Autodesk Fusion 360 part; units mm, degrees
(part 4 of 5)
  spline S202 degree 5 poles (32.0875, 34.5814) (32.0719, 34.5758) (32.0408, 34.5645) (31.9942, 34.5475) (31.9321, 34.5247) (31.8546, 34.496) (31.7774, 34.4669) (31.7004, 34.4376) (31.6235, 34.408) (31.5469, 34.3781) (31.4704, 34.348) (31.3942, 34.3176) (31.3181, 34.2869) (31.2423, 34.2559) (31.1666, 34.2246) (31.0912, 34.1931) (31.016, 34.1613) (30.941, 34.1291) (30.8662, 34.0967) (30.7916, 34.0641) (30.7172, 34.0311) (30.6563, 34.0037) (30.6103, 33.9829) (30.5792, 33.9687) (30.5628, 33.9613) (30.5612, 33.9605) knots -1 -1 -1 -1 -1 -1 -0.985714 -0.971429 -0.957143 -0.942857 -0.928571 -0.914286 -0.9 -0.885714 -0.871429 -0.857143 -0.842857 -0.828571 -0.814286 -0.8 -0.785714 -0.771429 -0.757143 -0.742857 -0.728571 -0.714286 -0.712736 -0.712736 -0.712736 -0.712736 -0.712736 -0.712736
  spline S203 degree 5 poles (-44.686, 9.5112) (-44.6878, 9.5109) (-44.7054, 9.5073) (-44.7389, 9.5005) (-44.7884, 9.4903) (-44.8537, 9.4766) (-44.9333, 9.4596) (-45.0128, 9.4422) (-45.0924, 9.4244) (-45.1719, 9.4063) (-45.2515, 9.3878) (-45.3311, 9.369) (-45.4106, 9.3498) (-45.4902, 9.3303) (-45.5698, 9.3105) (-45.6494, 9.2903) (-45.7289, 9.2697) (-45.8085, 9.2488) (-45.8881, 9.2276) (-45.9676, 9.206) (-46.0472, 9.1841) (-46.1267, 9.1619) (-46.1903, 9.1438) (-46.2381, 9.1301) (-46.2699, 9.121) (-46.2858, 9.1163) knots 0.712736 0.712736 0.712736 0.712736 0.712736 0.712736 0.714286 0.728571 0.742857 0.757143 0.771429 0.785714 0.8 0.814286 0.828571 0.842857 0.857143 0.871429 0.885714 0.9 0.914286 0.928571 0.942857 0.957143 0.971429 0.985714 1 1 1 1 1 1
  spline S204 degree 5 poles (-29.8528, -36.5279) (-29.8376, -36.5213) (-29.8073, -36.5081) (-29.7618, -36.4883) (-29.7012, -36.4616) (-29.6258, -36.4281) (-29.5505, -36.3942) (-29.4755, -36.3601) (-29.4006, -36.3258) (-29.326, -36.2911) (-29.2516, -36.2563) (-29.1774, -36.2211) (-29.1034, -36.1857) (-29.0297, -36.15) (-28.9562, -36.1141) (-28.8829, -36.0778) (-28.8098, -36.0414) (-28.7369, -36.0046) (-28.6643, -35.9676) (-28.5919, -35.9303) (-28.5198, -35.8927) (-28.4607, -35.8616) (-28.4161, -35.8379) (-28.3859, -35.8218) (-28.3701, -35.8133) (-28.3685, -35.8125) knots -1 -1 -1 -1 -1 -1 -0.985714 -0.971429 -0.957143 -0.942857 -0.928571 -0.914286 -0.9 -0.885714 -0.871429 -0.857143 -0.842857 -0.828571 -0.814286 -0.8 -0.785714 -0.771429 -0.757143 -0.742857 -0.728571 -0.714286 -0.712736 -0.712736 -0.712736 -0.712736 -0.712736 -0.712736
  spline S205 degree 3 poles (33.9605, 30.5612) (33.9329, 30.5008) (33.9173, 30.4356) (33.9121, 30.3029) (33.9225, 30.2367) (33.968, 30.1119) (34.0027, 30.0546) (34.0922, 29.9564) (34.1461, 29.9166) (34.2662, 29.8597) (34.3312, 29.8433) (34.4581, 29.8366) (34.5187, 29.8443) (34.5766, 29.8624) knots 0 0 0 0 0.019923 0.019923 0.039846 0.039846 0.059769 0.059769 0.079691 0.079691 0.099614 0.099614 0.117812 0.117812 0.117812 0.117812
  spline S206 degree 5 poles (-33.9605, -30.5612) (-33.9613, -30.5628) (-33.9687, -30.5792) (-33.9829, -30.6103) (-34.0037, -30.6563) (-34.0311, -30.7172) (-34.0641, -30.7916) (-34.0967, -30.8662) (-34.1291, -30.941) (-34.1613, -31.016) (-34.1931, -31.0912) (-34.2246, -31.1666) (-34.2559, -31.2423) (-34.2869, -31.3181) (-34.3176, -31.3942) (-34.348, -31.4704) (-34.3781, -31.5469) (-34.408, -31.6235) (-34.4376, -31.7004) (-34.4669, -31.7774) (-34.496, -31.8546) (-34.5247, -31.9321) (-34.5475, -31.9942) (-34.5645, -32.0408) (-34.5758, -32.0719) (-34.5814, -32.0875) knots 0.712736 0.712736 0.712736 0.712736 0.712736 0.712736 0.714286 0.728571 0.742857 0.757143 0.771429 0.785714 0.8 0.814286 0.828571 0.842857 0.857143 0.871429 0.885714 0.9 0.914286 0.928571 0.942857 0.957143 0.971429 0.985714 1 1 1 1 1 1
  line L71 (-17.6723, -23.7419) -> (-22.5976, -30.046)
  arc A132 (-25.5151, -39.6795) -> (-25.0393, -39.9814) centre (0, 0) ccw
  arc A133 (22.9733, 41.2033) -> (22.4794, 41.4748) centre (0, 0) ccw
  arc A134 (-36.5279, -29.8528) -> (-36.1687, -30.2871) centre (0, 0) ccw
  spline S207 degree 5 poles (34.1956, 32.4983) (34.1797, 32.4937) (34.1479, 32.4844) (34.1003, 32.4704) (34.0369, 32.4516) (33.9578, 32.4277) (33.8789, 32.4036) (33.8002, 32.3792) (33.7216, 32.3544) (33.6433, 32.3295) (33.5651, 32.3042) (33.4871, 32.2786) (33.4092, 32.2527) (33.3316, 32.2266) (33.2541, 32.2001) (33.1769, 32.1734) (33.0998, 32.1463) (33.0229, 32.119) (32.9462, 32.0914) (32.8697, 32.0634) (32.7934, 32.0352) (32.7309, 32.0117) (32.6837, 31.9938) (32.6518, 31.9816) (32.635, 31.9752) (32.6333, 31.9746) knots -1 -1 -1 -1 -1 -1 -0.985714 -0.971429 -0.957143 -0.942857 -0.928571 -0.914286 -0.9 -0.885714 -0.871429 -0.857143 -0.842857 -0.828571 -0.814286 -0.8 -0.785714 -0.771429 -0.757143 -0.742857 -0.728571 -0.714286 -0.712736 -0.712736 -0.712736 -0.712736 -0.712736 -0.712736
  spline S208 degree 5 poles (-25.0393, -39.9814) (-25.025, -39.973) (-24.9965, -39.9561) (-24.9539, -39.9307) (-24.8972, -39.8967) (-24.8265, -39.8539) (-24.7561, -39.8109) (-24.6859, -39.7677) (-24.616, -39.7242) (-24.5463, -39.6805) (-24.4768, -39.6366) (-24.4076, -39.5924) (-24.3387, -39.548) (-24.27, -39.5033) (-24.2015, -39.4585) (-24.1333, -39.4133) (-24.0654, -39.368) (-23.9978, -39.3224) (-23.9304, -39.2765) (-23.8632, -39.2305) (-23.7964, -39.1841) (-23.7416, -39.1459) (-23.7004, -39.1168) (-23.6724, -39.097) (-23.6578, -39.0866) (-23.6563, -39.0856) knots -1 -1 -1 -1 -1 -1 -0.985714 -0.971429 -0.957143 -0.942857 -0.928571 -0.914286 -0.9 -0.885714 -0.871429 -0.857143 -0.842857 -0.828571 -0.814286 -0.8 -0.785714 -0.771429 -0.757143 -0.742857 -0.728571 -0.714286 -0.712736 -0.712736 -0.712736 -0.712736 -0.712736 -0.712736
  spline S209 degree 5 poles (-21.1555, 40.4939) (-21.1568, 40.495) (-21.1708, 40.5063) (-21.1974, 40.5278) (-21.2368, 40.5594) (-21.289, 40.601) (-21.3528, 40.6514) (-21.4169, 40.7016) (-21.4813, 40.7516) (-21.546, 40.8014) (-21.6109, 40.8509) (-21.6762, 40.9002) (-21.7417, 40.9493) (-21.8074, 40.9982) (-21.8734, 41.0468) (-21.9397, 41.0953) (-22.0063, 41.1435) (-22.0731, 41.1915) (-22.1402, 41.2392) (-22.2075, 41.2868) (-22.2751, 41.3341) (-22.3429, 41.3812) (-22.3974, 41.4188) (-22.4383, 41.4468) (-22.4657, 41.4655) (-22.4794, 41.4748) knots 0.712736 0.712736 0.712736 0.712736 0.712736 0.712736 0.714286 0.728571 0.742857 0.757143 0.771429 0.785714 0.8 0.814286 0.828571 0.842857 0.857143 0.871429 0.885714 0.9 0.914286 0.928571 0.942857 0.957143 0.971429 0.985714 1 1 1 1 1 1
  spline S210 degree 5 poles (-28.3685, 35.8125) (-28.3701, 35.8133) (-28.3859, 35.8218) (-28.4161, 35.8379) (-28.4607, 35.8616) (-28.5198, 35.8927) (-28.5919, 35.9303) (-28.6643, 35.9676) (-28.7369, 36.0046) (-28.8098, 36.0414) (-28.8829, 36.0778) (-28.9562, 36.1141) (-29.0297, 36.15) (-29.1034, 36.1857) (-29.1774, 36.2211) (-29.2516, 36.2563) (-29.326, 36.2911) (-29.4006, 36.3258) (-29.4755, 36.3601) (-29.5505, 36.3942) (-29.6258, 36.4281) (-29.7012, 36.4616) (-29.7618, 36.4883) (-29.8073, 36.5081) (-29.8376, 36.5213) (-29.8528, 36.5279) knots 0.712736 0.712736 0.712736 0.712736 0.712736 0.712736 0.714286 0.728571 0.742857 0.757143 0.771429 0.785714 0.8 0.814286 0.828571 0.842857 0.857143 0.871429 0.885714 0.9 0.914286 0.928571 0.942857 0.957143 0.971429 0.985714 1 1 1 1 1 1
  arc A135 (-30.2871, -36.1687) -> (-29.8528, -36.5279) centre (0, 0) ccw
  spline S211 degree 5 poles (-32.0875, -34.5814) (-32.0719, -34.5758) (-32.0408, -34.5645) (-31.9942, -34.5475) (-31.9321, -34.5247) (-31.8546, -34.496) (-31.7774, -34.4669) (-31.7004, -34.4376) (-31.6235, -34.408) (-31.5469, -34.3781) (-31.4704, -34.348) (-31.3942, -34.3176) (-31.3181, -34.2869) (-31.2423, -34.2559) (-31.1666, -34.2246) (-31.0912, -34.1931) (-31.016, -34.1613) (-30.941, -34.1291) (-30.8662, -34.0967) (-30.7916, -34.0641) (-30.7172, -34.0311) (-30.6563, -34.0037) (-30.6103, -33.9829) (-30.5792, -33.9687) (-30.5628, -33.9613) (-30.5612, -33.9605) knots -1 -1 -1 -1 -1 -1 -0.985714 -0.971429 -0.957143 -0.942857 -0.928571 -0.914286 -0.9 -0.885714 -0.871429 -0.857143 -0.842857 -0.828571 -0.814286 -0.8 -0.785714 -0.771429 -0.757143 -0.742857 -0.728571 -0.714286 -0.712736 -0.712736 -0.712736 -0.712736 -0.712736 -0.712736
  arc A136 (-19.8308, 42.8044) -> (-20.3407, 42.5645) centre (0, 0) ccw
  spline S212 degree 5 poles (-36.1687, -30.2871) (-36.1525, -30.2834) (-36.1202, -30.2762) (-36.0718, -30.2652) (-36.0074, -30.2503) (-35.927, -30.2315) (-35.8467, -30.2124) (-35.7666, -30.1929) (-35.6866, -30.1732) (-35.6069, -30.1532) (-35.5272, -30.1329) (-35.4478, -30.1122) (-35.3685, -30.0913) (-35.2893, -30.0701) (-35.2104, -30.0485) (-35.1316, -30.0267) (-35.053, -30.0046) (-34.9745, -29.9821) (-34.8962, -29.9593) (-34.8182, -29.9362) (-34.7402, -29.9128) (-34.6764, -29.8934) (-34.6281, -29.8785) (-34.5955, -29.8683) (-34.5783, -29.8629) (-34.5766, -29.8624) knots -1 -1 -1 -1 -1 -1 -0.985714 -0.971429 -0.957143 -0.942857 -0.928571 -0.914286 -0.9 -0.885714 -0.871429 -0.857143 -0.842857 -0.828571 -0.814286 -0.8 -0.785714 -0.771429 -0.757143 -0.742857 -0.728571 -0.714286 -0.712736 -0.712736 -0.712736 -0.712736 -0.712736 -0.712736
  arc A137 (-44.7782, 14.8456) -> (-44.9524, 14.3096) centre (0, 0) ccw
  spline S213 degree 5 poles (-34.1956, -32.4983) (-34.1797, -32.4937) (-34.1479, -32.4844) (-34.1003, -32.4704) (-34.0369, -32.4516) (-33.9578, -32.4277) (-33.8789, -32.4036) (-33.8002, -32.3792) (-33.7216, -32.3544) (-33.6433, -32.3295) (-33.5651, -32.3042) (-33.4871, -32.2786) (-33.4092, -32.2527) (-33.3316, -32.2266) (-33.2541, -32.2001) (-33.1769, -32.1734) (-33.0998, -32.1463) (-33.0229, -32.119) (-32.9462, -32.0914) (-32.8697, -32.0634) (-32.7934, -32.0352) (-32.7309, -32.0117) (-32.6837, -31.9938) (-32.6518, -31.9816) (-32.635, -31.9752) (-32.6333, -31.9746) knots -1 -1 -1 -1 -1 -1 -0.985714 -0.971429 -0.957143 -0.942857 -0.928571 -0.914286 -0.9 -0.885714 -0.871429 -0.857143 -0.842857 -0.828571 -0.814286 -0.8 -0.785714 -0.771429 -0.757143 -0.742857 -0.728571 -0.714286 -0.712736 -0.712736 -0.712736 -0.712736 -0.712736 -0.712736
  arc A138 (32.4983, 34.1956) -> (32.0875, 34.5814) centre (0, 0) ccw
  spline S214 degree 3 poles (-33.9605, -30.5612) (-33.9329, -30.5008) (-33.9173, -30.4356) (-33.9121, -30.3029) (-33.9225, -30.2367) (-33.968, -30.1119) (-34.0027, -30.0546) (-34.0922, -29.9564) (-34.1461, -29.9166) (-34.2662, -29.8597) (-34.3312, -29.8433) (-34.4581, -29.8366) (-34.5187, -29.8443) (-34.5766, -29.8624) knots 0 0 0 0 0.019923 0.019923 0.039846 0.039846 0.059769 0.059769 0.079691 0.079691 0.099614 0.099614 0.117812 0.117812 0.117812 0.117812
  arc A139 (-24.2327, 28.4902) -> (-25.7909, 27.0472) centre (0.7975, -0.1016) ccw
  spline S215 degree 3 poles (-37.5231, -26.0639) (-37.4881, -26.0074) (-37.4645, -25.9447) (-37.4427, -25.8136) (-37.4446, -25.7466) (-37.4742, -25.6171) (-37.5014, -25.5559) (-37.5779, -25.4473) (-37.6264, -25.401) (-37.7384, -25.3296) (-37.8008, -25.3052) (-37.9259, -25.2826) (-37.987, -25.2826) (-38.0467, -25.2933) knots 0 0 0 0 0.019923 0.019923 0.039846 0.039846 0.059769 0.059769 0.079691 0.079691 0.099614 0.099614 0.117812 0.117812 0.117812 0.117812
  spline S216 degree 5 poles (29.8624, 34.5766) (29.8629, 34.5783) (29.8683, 34.5955) (29.8785, 34.6281) (29.8934, 34.6764) (29.9128, 34.7402) (29.9362, 34.8182) (29.9593, 34.8962) (29.9821, 34.9745) (30.0046, 35.053) (30.0267, 35.1316) (30.0485, 35.2104) (30.0701, 35.2893) (30.0913, 35.3685) (30.1122, 35.4478) (30.1329, 35.5272) (30.1532, 35.6069) (30.1732, 35.6866) (30.1929, 35.7666) (30.2124, 35.8467) (30.2315, 35.927) (30.2503, 36.0074) (30.2652, 36.0718) (30.2762, 36.1202) (30.2834, 36.1525) (30.2871, 36.1687) knots 0.712736 0.712736 0.712736 0.712736 0.712736 0.712736 0.714286 0.728571 0.742857 0.757143 0.771429 0.785714 0.8 0.814286 0.828571 0.842857 0.857143 0.871429 0.885714 0.9 0.914286 0.928571 0.942857 0.957143 0.971429 0.985714 1 1 1 1 1 1
  spline S217 degree 3 poles (-38.0467, 25.2933) (-37.9814, 25.2816) (-37.9143, 25.2827) (-37.7845, 25.3107) (-37.7229, 25.3372) (-37.6134, 25.4123) (-37.5665, 25.4602) (-37.4937, 25.5713) (-37.4685, 25.6334) (-37.4433, 25.7638) (-37.4436, 25.8309) (-37.4686, 25.9554) (-37.4911, 26.0123) (-37.5231, 26.0639) knots 0 0 0 0 0.019923 0.019923 0.039846 0.039846 0.059769 0.059769 0.079691 0.079691 0.099614 0.099614 0.117812 0.117812 0.117812 0.117812
  arc A140 (-25.0393, 39.9814) -> (-25.5151, 39.6795) centre (0, 0) ccw
  spline S218 degree 5 poles (-30.5612, 33.9605) (-30.5628, 33.9613) (-30.5792, 33.9687) (-30.6103, 33.9829) (-30.6563, 34.0037) (-30.7172, 34.0311) (-30.7916, 34.0641) (-30.8662, 34.0967) (-30.941, 34.1291) (-31.016, 34.1613) (-31.0912, 34.1931) (-31.1666, 34.2246) (-31.2423, 34.2559) (-31.3181, 34.2869) (-31.3942, 34.3176) (-31.4704, 34.348) (-31.5469, 34.3781) (-31.6235, 34.408) (-31.7004, 34.4376) (-31.7774, 34.4669) (-31.8546, 34.496) (-31.9321, 34.5247) (-31.9942, 34.5475) (-32.0408, 34.5645) (-32.0719, 34.5758) (-32.0875, 34.5814) knots 0.712736 0.712736 0.712736 0.712736 0.712736 0.712736 0.714286 0.728571 0.742857 0.757143 0.771429 0.785714 0.8 0.814286 0.828571 0.842857 0.857143 0.871429 0.885714 0.9 0.914286 0.928571 0.942857 0.957143 0.971429 0.985714 1 1 1 1 1 1
  spline S219 degree 3 poles (35.8125, 28.3685) (35.7811, 28.31) (35.7615, 28.2459) (35.7479, 28.1138) (35.7541, 28.047) (35.7917, 27.9196) (35.8228, 27.8602) (35.9059, 27.7566) (35.9572, 27.7135) (36.0735, 27.6492) (36.1373, 27.6288) (36.2635, 27.6141) (36.3246, 27.6179) (36.3835, 27.6324) knots 0 0 0 0 0.019923 0.019923 0.039846 0.039846 0.059769 0.059769 0.079691 0.079691 0.099614 0.099614 0.117812 0.117812 0.117812 0.117812
  spline S220 degree 5 poles (37.9991, 27.9562) (37.9827, 27.9536) (37.95, 27.9484) (37.901, 27.9405) (37.8358, 27.9297) (37.7543, 27.916) (37.673, 27.9019) (37.5918, 27.8875) (37.5108, 27.8729) (37.4299, 27.8579) (37.3492, 27.8426) (37.2686, 27.827) (37.1881, 27.8111) (37.1078, 27.7949) (37.0277, 27.7784) (36.9476, 27.7615) (36.8678, 27.7444) (36.7881, 27.7269) (36.7085, 27.7091) (36.6292, 27.6909) (36.5499, 27.6725) (36.485, 27.657) (36.4359, 27.6452) (36.4027, 27.6371) (36.3852, 27.6328) (36.3835, 27.6324) knots -1 -1 -1 -1 -1 -1 -0.985714 -0.971429 -0.957143 -0.942857 -0.928571 -0.914286 -0.9 -0.885714 -0.871429 -0.857143 -0.842857 -0.828571 -0.814286 -0.8 -0.785714 -0.771429 -0.757143 -0.742857 -0.728571 -0.714286 -0.712736 -0.712736 -0.712736 -0.712736 -0.712736 -0.712736
  spline S221 degree 3 poles (-32.6333, 31.9746) (-32.5713, 31.9508) (-32.5053, 31.9393) (-32.3725, 31.9424) (-32.307, 31.9569) (-32.1854, 32.0102) (-32.1303, 32.0485) (-32.038, 32.144) (-32.0016, 32.2003) (-31.9524, 32.3237) (-31.9401, 32.3896) (-31.9414, 32.5166) (-31.9528, 32.5767) (-31.9746, 32.6333) knots 0 0 0 0 0.019923 0.019923 0.039846 0.039846 0.059769 0.059769 0.079691 0.079691 0.099614 0.099614 0.117812 0.117812 0.117812 0.117812
  spline S222 degree 5 poles (-34.5766, 29.8624) (-34.5783, 29.8629) (-34.5955, 29.8683) (-34.6281, 29.8785) (-34.6764, 29.8934) (-34.7402, 29.9128) (-34.8182, 29.9362) (-34.8962, 29.9593) (-34.9745, 29.9821) (-35.053, 30.0046) (-35.1316, 30.0267) (-35.2104, 30.0485) (-35.2893, 30.0701) (-35.3685, 30.0913) (-35.4478, 30.1122) (-35.5272, 30.1329) (-35.6069, 30.1532) (-35.6866, 30.1732) (-35.7666, 30.1929) (-35.8467, 30.2124) (-35.927, 30.2315) (-36.0074, 30.2503) (-36.0718, 30.2652) (-36.1202, 30.2762) (-36.1525, 30.2834) (-36.1687, 30.2871) knots 0.712736 0.712736 0.712736 0.712736 0.712736 0.712736 0.714286 0.728571 0.742857 0.757143 0.771429 0.785714 0.8 0.814286 0.828571 0.842857 0.857143 0.871429 0.885714 0.9 0.914286 0.928571 0.942857 0.957143 0.971429 0.985714 1 1 1 1 1 1
  spline S223 degree 5 poles (-45.0493, -7.6067) (-45.0508, -7.6077) (-45.0659, -7.6175) (-45.0946, -7.6362) (-45.1368, -7.6639) (-45.1925, -7.7007) (-45.2602, -7.7458) (-45.3278, -7.7912) (-45.3952, -7.837) (-45.4625, -7.8831) (-45.5297, -7.9296) (-45.5967, -7.9764) (-45.6637, -8.0235) (-45.7305, -8.0709) (-45.7971, -8.1187) (-45.8637, -8.1668) (-45.9301, -8.2152) (-45.9964, -8.2639) (-46.0625, -8.3129) (-46.1286, -8.3623) (-46.1945, -8.4119) (-46.2602, -8.4619) (-46.3128, -8.5021) (-46.3521, -8.5324) (-46.3783, -8.5526) (-46.3914, -8.5628) knots 0.712736 0.712736 0.712736 0.712736 0.712736 0.712736 0.714286 0.728571 0.742857 0.757143 0.771429 0.785714 0.8 0.814286 0.828571 0.842857 0.857143 0.871429 0.885714 0.9 0.914286 0.928571 0.942857 0.957143 0.971429 0.985714 1 1 1 1 1 1
  arc A141 (30.2871, 36.1687) -> (29.8528, 36.5279) centre (0, 0) ccw
  arc A142 (36.5279, 29.8528) -> (36.1687, 30.2871) centre (0, 0) ccw
  arc A143 (-32.0875, 34.5814) -> (-32.4983, 34.1956) centre (0, 0) ccw
  arc A144 (38.3303, 27.5003) -> (37.9991, 27.9562) centre (0, 0) ccw
  arc A145 (-36.1687, 30.2871) -> (-36.5279, 29.8528) centre (0, 0) ccw
  spline S224 degree 5 poles (-30.2871, 36.1687) (-30.2834, 36.1525) (-30.2762, 36.1202) (-30.2652, 36.0718) (-30.2503, 36.0074) (-30.2315, 35.927) (-30.2124, 35.8467) (-30.1929, 35.7666) (-30.1732, 35.6866) (-30.1532, 35.6069) (-30.1329, 35.5272) (-30.1122, 35.4478) (-30.0913, 35.3685) (-30.0701, 35.2893) (-30.0485, 35.2104) (-30.0267, 35.1316) (-30.0046, 35.053) (-29.9821, 34.9745) (-29.9593, 34.8962) (-29.9362, 34.8182) (-29.9128, 34.7402) (-29.8934, 34.6764) (-29.8785, 34.6281) (-29.8683, 34.5955) (-29.8629, 34.5783) (-29.8624, 34.5766) knots -1 -1 -1 -1 -1 -1 -0.985714 -0.971429 -0.957143 -0.942857 -0.928571 -0.914286 -0.9 -0.885714 -0.871429 -0.857143 -0.842857 -0.828571 -0.814286 -0.8 -0.785714 -0.771429 -0.757143 -0.742857 -0.728571 -0.714286 -0.712736 -0.712736 -0.712736 -0.712736 -0.712736 -0.712736
  spline S225 degree 5 poles (-27.9562, 37.9991) (-27.9536, 37.9827) (-27.9484, 37.95) (-27.9405, 37.901) (-27.9297, 37.8358) (-27.916, 37.7543) (-27.9019, 37.673) (-27.8875, 37.5918) (-27.8729, 37.5108) (-27.8579, 37.4299) (-27.8426, 37.3492) (-27.827, 37.2686) (-27.8111, 37.1881) (-27.7949, 37.1078) (-27.7784, 37.0277) (-27.7615, 36.9476) (-27.7444, 36.8678) (-27.7269, 36.7881) (-27.7091, 36.7085) (-27.6909, 36.6292) (-27.6725, 36.5499) (-27.657, 36.485) (-27.6452, 36.4359) (-27.6371, 36.4027) (-27.6328, 36.3852) (-27.6324, 36.3835) knots -1 -1 -1 -1 -1 -1 -0.985714 -0.971429 -0.957143 -0.942857 -0.928571 -0.914286 -0.9 -0.885714 -0.871429 -0.857143 -0.842857 -0.828571 -0.814286 -0.8 -0.785714 -0.771429 -0.757143 -0.742857 -0.728571 -0.714286 -0.712736 -0.712736 -0.712736 -0.712736 -0.712736 -0.712736
  line L72 (-21.8014, -19.8321) -> (-27.9672, -24.9329)
  spline S226 degree 5 poles (-36.5279, 29.8528) (-36.5213, 29.8376) (-36.5081, 29.8073) (-36.4883, 29.7618) (-36.4616, 29.7012) (-36.4281, 29.6258) (-36.3942, 29.5505) (-36.3601, 29.4755) (-36.3258, 29.4006) (-36.2911, 29.326) (-36.2563, 29.2516) (-36.2211, 29.1774) (-36.1857, 29.1034) (-36.15, 29.0297) (-36.1141, 28.9562) (-36.0778, 28.8829) (-36.0414, 28.8098) (-36.0046, 28.7369) (-35.9676, 28.6643) (-35.9303, 28.5919) (-35.8927, 28.5198) (-35.8616, 28.4607) (-35.8379, 28.4161) (-35.8218, 28.3859) (-35.8133, 28.3701) (-35.8125, 28.3685) knots -1 -1 -1 -1 -1 -1 -0.985714 -0.971429 -0.957143 -0.942857 -0.928571 -0.914286 -0.9 -0.885714 -0.871429 -0.857143 -0.842857 -0.828571 -0.814286 -0.8 -0.785714 -0.771429 -0.757143 -0.742857 -0.728571 -0.714286 -0.712736 -0.712736 -0.712736 -0.712736 -0.712736 -0.712736
  spline S227 degree 3 poles (-36.3835, 27.6324) (-36.319, 27.6166) (-36.252, 27.6135) (-36.1207, 27.6332) (-36.0575, 27.6558) (-35.9435, 27.7239) (-35.8937, 27.7688) (-35.8141, 27.8751) (-35.785, 27.9355) (-35.7517, 28.0641) (-35.7477, 28.131) (-35.7649, 28.2569) (-35.7838, 28.3151) (-35.8125, 28.3685) knots 0 0 0 0 0.019923 0.019923 0.039846 0.039846 0.059769 0.059769 0.079691 0.079691 0.099614 0.099614 0.117812 0.117812 0.117812 0.117812
  line L73 (-28.5113, -6.5044) -> (-36.3717, -8.0039)
  spline S228 degree 5 poles (31.9746, 32.6333) (31.9752, 32.635) (31.9816, 32.6518) (31.9938, 32.6837) (32.0117, 32.7309) (32.0352, 32.7934) (32.0634, 32.8697) (32.0914, 32.9462) (32.119, 33.0229) (32.1463, 33.0998) (32.1734, 33.1769) (32.2001, 33.2541) (32.2266, 33.3316) (32.2527, 33.4092) (32.2786, 33.4871) (32.3042, 33.5651) (32.3295, 33.6433) (32.3544, 33.7216) (32.3792, 33.8002) (32.4036, 33.8789) (32.4277, 33.9578) (32.4516, 34.0369) (32.4704, 34.1003) (32.4844, 34.1479) (32.4937, 34.1797) (32.4983, 34.1956) knots 0.712736 0.712736 0.712736 0.712736 0.712736 0.712736 0.714286 0.728571 0.742857 0.757143 0.771429 0.785714 0.8 0.814286 0.828571 0.842857 0.857143 0.871429 0.885714 0.9 0.914286 0.928571 0.942857 0.957143 0.971429 0.985714 1 1 1 1 1 1
  arc A146 (-17.6723, -23.7419) -> (-16.1846, -24.8323) centre (0.7975, -0.1016) ccw
  spline S229 degree 5 poles (-36.3835, 27.6324) (-36.3852, 27.6328) (-36.4027, 27.6371) (-36.4359, 27.6452) (-36.485, 27.657) (-36.5499, 27.6725) (-36.6292, 27.6909) (-36.7085, 27.7091) (-36.7881, 27.7269) (-36.8678, 27.7444) (-36.9476, 27.7615) (-37.0277, 27.7784) (-37.1078, 27.7949) (-37.1881, 27.8111) (-37.2686, 27.827) (-37.3492, 27.8426) (-37.4299, 27.8579) (-37.5108, 27.8729) (-37.5918, 27.8875) (-37.673, 27.9019) (-37.7543, 27.916) (-37.8358, 27.9297) (-37.901, 27.9405) (-37.95, 27.9484) (-37.9827, 27.9536) (-37.9991, 27.9562) knots 0.712736 0.712736 0.712736 0.712736 0.712736 0.712736 0.714286 0.728571 0.742857 0.757143 0.771429 0.785714 0.8 0.814286 0.828571 0.842857 0.857143 0.871429 0.885714 0.9 0.914286 0.928571 0.942857 0.957143 0.971429 0.985714 1 1 1 1 1 1
  spline S230 degree 5 poles (-22.4794, -41.4748) (-22.4657, -41.4655) (-22.4383, -41.4468) (-22.3974, -41.4188) (-22.3429, -41.3812) (-22.2751, -41.3341) (-22.2075, -41.2868) (-22.1402, -41.2392) (-22.0731, -41.1915) (-22.0063, -41.1435) (-21.9397, -41.0953) (-21.8734, -41.0468) (-21.8074, -40.9982) (-21.7417, -40.9493) (-21.6762, -40.9002) (-21.6109, -40.8509) (-21.546, -40.8014) (-21.4813, -40.7516) (-21.4169, -40.7016) (-21.3528, -40.6514) (-21.289, -40.601) (-21.2368, -40.5594) (-21.1974, -40.5278) (-21.1708, -40.5063) (-21.1568, -40.495) (-21.1555, -40.4939) knots -1 -1 -1 -1 -1 -1 -0.985714 -0.971429 -0.957143 -0.942857 -0.928571 -0.914286 -0.9 -0.885714 -0.871429 -0.857143 -0.842857 -0.828571 -0.814286 -0.8 -0.785714 -0.771429 -0.757143 -0.742857 -0.728571 -0.714286 -0.712736 -0.712736 -0.712736 -0.712736 -0.712736 -0.712736
  arc A147 (-29.8528, 36.5279) -> (-30.2871, 36.1687) centre (0, 0) ccw
  line L74 (-25.0779, -15.2826) -> (-31.978, -19.3309)
  arc A148 (-20.4896, -21.2406) -> (-19.1503, -22.5089) centre (0.7975, -0.1016) ccw
  spline S231 degree 5 poles (-23.6563, 39.0856) (-23.6578, 39.0866) (-23.6724, 39.097) (-23.7004, 39.1168) (-23.7416, 39.1459) (-23.7964, 39.1841) (-23.8632, 39.2305) (-23.9304, 39.2765) (-23.9978, 39.3224) (-24.0654, 39.368) (-24.1333, 39.4133) (-24.2015, 39.4585) (-24.27, 39.5033) (-24.3387, 39.548) (-24.4076, 39.5924) (-24.4768, 39.6366) (-24.5463, 39.6805) (-24.616, 39.7242) (-24.6859, 39.7677) (-24.7561, 39.8109) (-24.8265, 39.8539) (-24.8972, 39.8967) (-24.9539, 39.9307) (-24.9965, 39.9561) (-25.025, 39.973) (-25.0393, 39.9814) knots 0.712736 0.712736 0.712736 0.712736 0.712736 0.712736 0.714286 0.728571 0.742857 0.757143 0.771429 0.785714 0.8 0.814286 0.828571 0.842857 0.857143 0.871429 0.885714 0.9 0.914286 0.928571 0.942857 0.957143 0.971429 0.985714 1 1 1 1 1 1
  spline S232 degree 3 poles (-34.5766, 29.8624) (-34.5132, 29.8426) (-34.4466, 29.8353) (-34.3143, 29.8467) (-34.2499, 29.8653) (-34.1318, 29.9261) (-34.0792, 29.9678) (-33.9931, 30.0689) (-33.9603, 30.1273) (-33.919, 30.2536) (-33.9108, 30.3201) (-33.9201, 30.4468) (-33.9353, 30.5061) (-33.9605, 30.5612) knots 0 0 0 0 0.019923 0.019923 0.039846 0.039846 0.059769 0.059769 0.079691 0.079691 0.099614 0.099614 0.117812 0.117812 0.117812 0.117812
  line L75 (-29.1908, -0.9393) -> (-37.1877, -1.1626)
  arc A149 (-28.0403, -8.3707) -> (-27.4777, -10.1273) centre (0.7975, -0.1016) ccw
  arc A150 (-28.8493, -4.6912) -> (-28.5113, -6.5044) centre (0.7975, -0.1016) ccw
  spline S233 degree 3 poles (-21.1555, 40.4939) (-21.1038, 40.4521) (-21.0445, 40.4208) (-20.9173, 40.3827) (-20.8506, 40.3763) (-20.7184, 40.3894) (-20.6542, 40.4087) (-20.5369, 40.471) (-20.4849, 40.5133) (-20.4, 40.6155) (-20.3679, 40.6743) (-20.3299, 40.7956) (-20.3222, 40.8562) (-20.3254, 40.9168) knots 0 0 0 0 0.019923 0.019923 0.039846 0.039846 0.059769 0.059769 0.079691 0.079691 0.099614 0.099614 0.117812 0.117812 0.117812 0.117812
  arc A151 (-25.0779, -15.2826) -> (-24.096, -16.8441) centre (0.7975, -0.1016) ccw
  spline S234 degree 5 poles (-22.9733, 41.2033) (-22.9727, 41.1867) (-22.9716, 41.1536) (-22.9699, 41.104) (-22.9674, 41.0379) (-22.964, 40.9554) (-22.9602, 40.873) (-22.9561, 40.7907) (-22.9517, 40.7084) (-22.947, 40.6263) (-22.942, 40.5443) (-22.9366, 40.4624) (-22.9309, 40.3805) (-22.9249, 40.2988) (-22.9185, 40.2172) (-22.9118, 40.1357) (-22.9048, 40.0544) (-22.8975, 39.9731) (-22.8898, 39.892) (-22.8817, 39.8109) (-22.8733, 39.73) (-22.8662, 39.6636) (-22.8606, 39.6135) (-22.8567, 39.5795) (-22.8546, 39.5616) (-22.8544, 39.5598) knots -1 -1 -1 -1 -1 -1 -0.985714 -0.971429 -0.957143 -0.942857 -0.928571 -0.914286 -0.9 -0.885714 -0.871429 -0.857143 -0.842857 -0.828571 -0.814286 -0.8 -0.785714 -0.771429 -0.757143 -0.742857 -0.728571 -0.714286 -0.712736 -0.712736 -0.712736 -0.712736 -0.712736 -0.712736
  spline S235 degree 5 poles (-44.4828, -10.4204) (-44.4842, -10.4215) (-44.4987, -10.4322) (-44.5261, -10.4526) (-44.5665, -10.4829) (-44.6198, -10.5231) (-44.6845, -10.5724) (-44.7491, -10.622) (-44.8135, -10.6719) (-44.8778, -10.7222) (-44.9419, -10.7728) (-45.0059, -10.8237) (-45.0698, -10.8749) (-45.1334, -10.9265) (-45.197, -10.9783) (-45.2604, -11.0305) (-45.3236, -11.083) (-45.3867, -11.1357) (-45.4497, -11.1888) (-45.5125, -11.2422) (-45.5751, -11.2959) (-45.6376, -11.3499) (-45.6875, -11.3933) (-45.7249, -11.426) (-45.7497, -11.4479) (-45.7622, -11.4588) knots 0.712736 0.712736 0.712736 0.712736 0.712736 0.712736 0.714286 0.728571 0.742857 0.757143 0.771429 0.785714 0.8 0.814286 0.828571 0.842857 0.857143 0.871429 0.885714 0.9 0.914286 0.928571 0.942857 0.957143 0.971429 0.985714 1 1 1 1 1 1
  spline S236 degree 5 poles (-46.2858, -9.1163) (-46.2699, -9.121) (-46.2381, -9.1301) (-46.1903, -9.1438) (-46.1267, -9.1619) (-46.0472, -9.1841) (-45.9676, -9.206) (-45.8881, -9.2276) (-45.8085, -9.2488) (-45.7289, -9.2697) (-45.6494, -9.2903) (-45.5698, -9.3105) (-45.4902, -9.3303) (-45.4106, -9.3498) (-45.3311, -9.369) (-45.2515, -9.3878) (-45.1719, -9.4063) (-45.0924, -9.4244) (-45.0128, -9.4422) (-44.9333, -9.4596) (-44.8537, -9.4766) (-44.7884, -9.4903) (-44.7389, -9.5005) (-44.7054, -9.5073) (-44.6878, -9.5109) (-44.686, -9.5112) knots -1 -1 -1 -1 -1 -1 -0.985714 -0.971429 -0.957143 -0.942857 -0.928571 -0.914286 -0.9 -0.885714 -0.871429 -0.857143 -0.842857 -0.828571 -0.814286 -0.8 -0.785714 -0.771429 -0.757143 -0.742857 -0.728571 -0.714286 -0.712736 -0.712736 -0.712736 -0.712736 -0.712736 -0.712736
  spline S237 degree 3 poles (29.8624, 34.5766) (29.8426, 34.5132) (29.8353, 34.4466) (29.8467, 34.3143) (29.8653, 34.2499) (29.9261, 34.1318) (29.9678, 34.0792) (30.0689, 33.9931) (30.1273, 33.9603) (30.2536, 33.919) (30.3201, 33.9108) (30.4468, 33.9201) (30.5061, 33.9353) (30.5612, 33.9605) knots 0 0 0 0 0.019923 0.019923 0.039846 0.039846 0.059769 0.059769 0.079691 0.079691 0.099614 0.099614 0.117812 0.117812 0.117812 0.117812
  spline S238 degree 5 poles (-41.2033, -22.9733) (-41.1867, -22.9727) (-41.1536, -22.9716) (-41.104, -22.9699) (-41.0379, -22.9674) (-40.9554, -22.964) (-40.873, -22.9602) (-40.7907, -22.9561) (-40.7084, -22.9517) (-40.6263, -22.947) (-40.5443, -22.942) (-40.4624, -22.9366) (-40.3805, -22.9309) (-40.2988, -22.9249) (-40.2172, -22.9185) (-40.1357, -22.9118) (-40.0544, -22.9048) (-39.9731, -22.8975) (-39.892, -22.8898) (-39.8109, -22.8817) (-39.73, -22.8733) (-39.6636, -22.8662) (-39.6135, -22.8606) (-39.5795, -22.8567) (-39.5616, -22.8546) (-39.5598, -22.8544) knots -1 -1 -1 -1 -1 -1 -0.985714 -0.971429 -0.957143 -0.942857 -0.928571 -0.914286 -0.9 -0.885714 -0.871429 -0.857143 -0.842857 -0.828571 -0.814286 -0.8 -0.785714 -0.771429 -0.757143 -0.742857 -0.728571 -0.714286 -0.712736 -0.712736 -0.712736 -0.712736 -0.712736 -0.712736
  arc A152 (-34.1956, 32.4983) -> (-34.5814, 32.0875) centre (0, 0) ccw
  spline S239 degree 3 poles (-40.4939, -21.1555) (-40.4521, -21.1038) (-40.4208, -21.0445) (-40.3827, -20.9173) (-40.3763, -20.8506) (-40.3894, -20.7184) (-40.4087, -20.6542) (-40.471, -20.5369) (-40.5133, -20.4849) (-40.6155, -20.4) (-40.6743, -20.3679) (-40.7956, -20.3299) (-40.8562, -20.3222) (-40.9168, -20.3254) knots 0 0 0 0 0.019923 0.019923 0.039846 0.039846 0.059769 0.059769 0.079691 0.079691 0.099614 0.099614 0.117812 0.117812 0.117812 0.117812
  spline S240 degree 5 poles (-38.3303, 27.5003) (-38.3228, 27.4856) (-38.3077, 27.4561) (-38.285, 27.4119) (-38.2546, 27.3532) (-38.2164, 27.28) (-38.1779, 27.207) (-38.1392, 27.1342) (-38.1002, 27.0617) (-38.0609, 26.9894) (-38.0214, 26.9173) (-37.9817, 26.8455) (-37.9417, 26.7739) (-37.9015, 26.7025) (-37.861, 26.6314) (-37.8202, 26.5605) (-37.7792, 26.4899) (-37.738, 26.4195) (-37.6964, 26.3493) (-37.6547, 26.2794) (-37.6126, 26.2098) (-37.5779, 26.1528) (-37.5514, 26.1098) (-37.5335, 26.0807) (-37.524, 26.0654) (-37.5231, 26.0639) knots -1 -1 -1 -1 -1 -1 -0.985714 -0.971429 -0.957143 -0.942857 -0.928571 -0.914286 -0.9 -0.885714 -0.871429 -0.857143 -0.842857 -0.828571 -0.814286 -0.8 -0.785714 -0.771429 -0.757143 -0.742857 -0.728571 -0.714286 -0.712736 -0.712736 -0.712736 -0.712736 -0.712736 -0.712736
  spline S241 degree 5 poles (-38.0467, 25.2933) (-38.0485, 25.2936) (-38.0662, 25.2968) (-38.0999, 25.3028) (-38.1496, 25.3115) (-38.2154, 25.3229) (-38.2956, 25.3363) (-38.376, 25.3494) (-38.4565, 25.3622) (-38.5371, 25.3747) (-38.6179, 25.3868) (-38.6988, 25.3986) (-38.7798, 25.41) (-38.861, 25.4212) (-38.9423, 25.432) (-39.0237, 25.4425) (-39.1053, 25.4527) (-39.1869, 25.4626) (-39.2687, 25.4721) (-39.3506, 25.4813) (-39.4327, 25.4903) (-39.5148, 25.4989) (-39.5806, 25.5055) (-39.63, 25.5104) (-39.663, 25.5135) (-39.6795, 25.5151) knots 0.712736 0.712736 0.712736 0.712736 0.712736 0.712736 0.714286 0.728571 0.742857 0.757143 0.771429 0.785714 0.8 0.814286 0.828571 0.842857 0.857143 0.871429 0.885714 0.9 0.914286 0.928571 0.942857 0.957143 0.971429 0.985714 1 1 1 1 1 1
  spline S242 degree 5 poles (-34.5814, 32.0875) (-34.5758, 32.0719) (-34.5645, 32.0408) (-34.5475, 31.9942) (-34.5247, 31.9321) (-34.496, 31.8546) (-34.4669, 31.7774) (-34.4376, 31.7004) (-34.408, 31.6235) (-34.3781, 31.5469) (-34.348, 31.4704) (-34.3176, 31.3942) (-34.2869, 31.3181) (-34.2559, 31.2423) (-34.2246, 31.1666) (-34.1931, 31.0912) (-34.1613, 31.016) (-34.1291, 30.941) (-34.0967, 30.8662) (-34.0641, 30.7916) (-34.0311, 30.7172) (-34.0037, 30.6563) (-33.9829, 30.6103) (-33.9687, 30.5792) (-33.9613, 30.5628) (-33.9605, 30.5612) knots -1 -1 -1 -1 -1 -1 -0.985714 -0.971429 -0.957143 -0.942857 -0.928571 -0.914286 -0.9 -0.885714 -0.871429 -0.857143 -0.842857 -0.828571 -0.814286 -0.8 -0.785714 -0.771429 -0.757143 -0.742857 -0.728571 -0.714286 -0.712736 -0.712736 -0.712736 -0.712736 -0.712736 -0.712736
  arc A153 (-39.6795, 25.5151) -> (-39.9814, 25.0393) centre (0, 0) ccw
  spline S243 degree 3 poles (-44.4828, -10.4204) (-44.4295, -10.3808) (-44.3845, -10.3311) (-44.3159, -10.2174) (-44.2931, -10.1543) (-44.2729, -10.0231) (-44.2757, -9.9561) (-44.3069, -9.827) (-44.3349, -9.7661) (-44.4127, -9.6584) (-44.4618, -9.6127) (-44.5698, -9.5457) (-44.6266, -9.5232) (-44.686, -9.5112) knots 0 0 0 0 0.019923 0.019923 0.039846 0.039846 0.059769 0.059769 0.079691 0.079691 0.099614 0.099614 0.117812 0.117812 0.117812 0.117812
  spline S244 degree 5 poles (33.9605, 30.5612) (33.9613, 30.5628) (33.9687, 30.5792) (33.9829, 30.6103) (34.0037, 30.6563) (34.0311, 30.7172) (34.0641, 30.7916) (34.0967, 30.8662) (34.1291, 30.941) (34.1613, 31.016) (34.1931, 31.0912) (34.2246, 31.1666) (34.2559, 31.2423) (34.2869, 31.3181) (34.3176, 31.3942) (34.348, 31.4704) (34.3781, 31.5469) (34.408, 31.6235) (34.4376, 31.7004) (34.4669, 31.7774) (34.496, 31.8546) (34.5247, 31.9321) (34.5475, 31.9942) (34.5645, 32.0408) (34.5758, 32.0719) (34.5814, 32.0875) knots 0.712736 0.712736 0.712736 0.712736 0.712736 0.712736 0.714286 0.728571 0.742857 0.757143 0.771429 0.785714 0.8 0.814286 0.828571 0.842857 0.857143 0.871429 0.885714 0.9 0.914286 0.928571 0.942857 0.957143 0.971429 0.985714 1 1 1 1 1 1
  spline S245 degree 5 poles (-39.0856, -23.6563) (-39.0866, -23.6578) (-39.097, -23.6724) (-39.1168, -23.7004) (-39.1459, -23.7416) (-39.1841, -23.7964) (-39.2305, -23.8632) (-39.2765, -23.9304) (-39.3224, -23.9978) (-39.368, -24.0654) (-39.4133, -24.1333) (-39.4585, -24.2015) (-39.5033, -24.27) (-39.548, -24.3387) (-39.5924, -24.4076) (-39.6366, -24.4768) (-39.6805, -24.5463) (-39.7242, -24.616) (-39.7677, -24.6859) (-39.8109, -24.7561) (-39.8539, -24.8265) (-39.8967, -24.8972) (-39.9307, -24.9539) (-39.9561, -24.9965) (-39.973, -25.025) (-39.9814, -25.0393) knots 0.712736 0.712736 0.712736 0.712736 0.712736 0.712736 0.714286 0.728571 0.742857 0.757143 0.771429 0.785714 0.8 0.814286 0.828571 0.842857 0.857143 0.871429 0.885714 0.9 0.914286 0.928571 0.942857 0.957143 0.971429 0.985714 1 1 1 1 1 1
  arc A154 (-47.0988, -2.6809) -> (-47.0634, -3.2433) centre (0, 0) ccw
  spline S246 degree 3 poles (37.5231, 26.0639) (37.4881, 26.0074) (37.4645, 25.9447) (37.4427, 25.8136) (37.4446, 25.7466) (37.4742, 25.6171) (37.5014, 25.5559) (37.5779, 25.4473) (37.6264, 25.401) (37.7384, 25.3296) (37.8008, 25.3052) (37.9259, 25.2826) (37.987, 25.2826) (38.0467, 25.2933) knots 0 0 0 0 0.019923 0.019923 0.039846 0.039846 0.059769 0.059769 0.079691 0.079691 0.099614 0.099614 0.117812 0.117812 0.117812 0.117812
  spline S247 degree 3 poles (-30.5612, 33.9605) (-30.5008, 33.9329) (-30.4356, 33.9173) (-30.3029, 33.9121) (-30.2367, 33.9225) (-30.1119, 33.968) (-30.0546, 34.0027) (-29.9564, 34.0922) (-29.9166, 34.1461) (-29.8597, 34.2662) (-29.8433, 34.3312) (-29.8366, 34.4581) (-29.8443, 34.5187) (-29.8624, 34.5766) knots 0 0 0 0 0.019923 0.019923 0.039846 0.039846 0.059769 0.059769 0.079691 0.079691 0.099614 0.099614 0.117812 0.117812 0.117812 0.117812
  spline S248 degree 5 poles (-25.5151, 39.6795) (-25.5135, 39.663) (-25.5104, 39.63) (-25.5055, 39.5806) (-25.4989, 39.5148) (-25.4903, 39.4327) (-25.4813, 39.3506) (-25.4721, 39.2687) (-25.4626, 39.1869) (-25.4527, 39.1053) (-25.4425, 39.0237) (-25.432, 38.9423) (-25.4212, 38.861) (-25.41, 38.7798) (-25.3986, 38.6988) (-25.3868, 38.6179) (-25.3747, 38.5371) (-25.3622, 38.4565) (-25.3494, 38.376) (-25.3363, 38.2956) (-25.3229, 38.2154) (-25.3115, 38.1496) (-25.3028, 38.0999) (-25.2968, 38.0662) (-25.2936, 38.0485) (-25.2933, 38.0467) knots -1 -1 -1 -1 -1 -1 -0.985714 -0.971429 -0.957143 -0.942857 -0.928571 -0.914286 -0.9 -0.885714 -0.871429 -0.857143 -0.842857 -0.828571 -0.814286 -0.8 -0.785714 -0.771429 -0.757143 -0.742857 -0.728571 -0.714286 -0.712736 -0.712736 -0.712736 -0.712736 -0.712736 -0.712736
  spline S249 degree 5 poles (-32.4983, 34.1956) (-32.4937, 34.1797) (-32.4844, 34.1479) (-32.4704, 34.1003) (-32.4516, 34.0369) (-32.4277, 33.9578) (-32.4036, 33.8789) (-32.3792, 33.8002) (-32.3544, 33.7216) (-32.3295, 33.6433) (-32.3042, 33.5651) (-32.2786, 33.4871) (-32.2527, 33.4092) (-32.2266, 33.3316) (-32.2001, 33.2541) (-32.1734, 33.1769) (-32.1463, 33.0998) (-32.119, 33.0229) (-32.0914, 32.9462) (-32.0634, 32.8697) (-32.0352, 32.7934) (-32.0117, 32.7309) (-31.9938, 32.6837) (-31.9816, 32.6518) (-31.9752, 32.635) (-31.9746, 32.6333) knots -1 -1 -1 -1 -1 -1 -0.985714 -0.971429 -0.957143 -0.942857 -0.928571 -0.914286 -0.9 -0.885714 -0.871429 -0.857143 -0.842857 -0.828571 -0.814286 -0.8 -0.785714 -0.771429 -0.757143 -0.742857 -0.728571 -0.714286 -0.712736 -0.712736 -0.712736 -0.712736 -0.712736 -0.712736
  spline S250 degree 5 poles (-32.6333, 31.9746) (-32.635, 31.9752) (-32.6518, 31.9816) (-32.6837, 31.9938) (-32.7309, 32.0117) (-32.7934, 32.0352) (-32.8697, 32.0634) (-32.9462, 32.0914) (-33.0229, 32.119) (-33.0998, 32.1463) (-33.1769, 32.1734) (-33.2541, 32.2001) (-33.3316, 32.2266) (-33.4092, 32.2527) (-33.4871, 32.2786) (-33.5651, 32.3042) (-33.6433, 32.3295) (-33.7216, 32.3544) (-33.8002, 32.3792) (-33.8789, 32.4036) (-33.9578, 32.4277) (-34.0369, 32.4516) (-34.1003, 32.4704) (-34.1479, 32.4844) (-34.1797, 32.4937) (-34.1956, 32.4983) knots 0.712736 0.712736 0.712736 0.712736 0.712736 0.712736 0.714286 0.728571 0.742857 0.757143 0.771429 0.785714 0.8 0.814286 0.828571 0.842857 0.857143 0.871429 0.885714 0.9 0.914286 0.928571 0.942857 0.957143 0.971429 0.985714 1 1 1 1 1 1
  arc A155 (-22.5976, -30.046) -> (-20.8882, -31.3062) centre (0.7975, -0.1016) ccw
  arc A156 (-22.4794, 41.4748) -> (-22.9733, 41.2033) centre (0, 0) ccw
  arc A157 (-37.9991, 27.9562) -> (-38.3303, 27.5003) centre (0, 0) ccw
  spline S251 degree 5 poles (-20.3407, 42.5645) (-20.3413, 42.5479) (-20.3422, 42.5148) (-20.3436, 42.4652) (-20.3453, 42.3991) (-20.347, 42.3165) (-20.3485, 42.234) (-20.3496, 42.1516) (-20.3504, 42.0693) (-20.3508, 41.987) (-20.3509, 41.9048) (-20.3507, 41.8227) (-20.3502, 41.7407) (-20.3493, 41.6588) (-20.3481, 41.5769) (-20.3465, 41.4952) (-20.3446, 41.4135) (-20.3423, 41.332) (-20.3398, 41.2505) (-20.3368, 41.1691) (-20.3335, 41.0878) (-20.3305, 41.0211) (-20.3281, 40.9707) (-20.3264, 40.9365) (-20.3254, 40.9186) (-20.3254, 40.9168) knots -1 -1 -1 -1 -1 -1 -0.985714 -0.971429 -0.957143 -0.942857 -0.928571 -0.914286 -0.9 -0.885714 -0.871429 -0.857143 -0.842857 -0.828571 -0.814286 -0.8 -0.785714 -0.771429 -0.757143 -0.742857 -0.728571 -0.714286 -0.712736 -0.712736 -0.712736 -0.712736 -0.712736 -0.712736
  spline S252 degree 3 poles (-23.6563, 39.0856) (-23.6022, 39.0471) (-23.541, 39.0196) (-23.4117, 38.9896) (-23.3447, 38.9874) (-23.2136, 39.0087) (-23.1507, 39.0321) (-23.0376, 39.1016) (-22.9883, 39.1471) (-22.91, 39.2544) (-22.8817, 39.3152) (-22.8514, 39.4386) (-22.8475, 39.4996) (-22.8544, 39.5598) knots 0 0 0 0 0.019923 0.019923 0.039846 0.039846 0.059769 0.059769 0.079691 0.079691 0.099614 0.099614 0.117812 0.117812 0.117812 0.117812
  arc A158 (39.9814, 25.0393) -> (39.6795, 25.5151) centre (0, 0) ccw
  arc A159 (-35.7304, -10.5758) -> (-35.0882, -12.6001) centre (0.7975, -0.1016) ccw
  arc A160 (-22.9712, -18.406) -> (-21.8014, -19.8321) centre (0.7975, -0.1016) ccw
  spline S253 degree 3 poles (-43.7407, -13.1929) (-43.69, -13.1501) (-43.6482, -13.0977) (-43.5869, -12.9798) (-43.5681, -12.9155) (-43.5562, -12.7832) (-43.5632, -12.7165) (-43.6024, -12.5896) (-43.6342, -12.5306) (-43.7186, -12.4281) (-43.7704, -12.3855) (-43.8824, -12.3255) (-43.9406, -12.3066) (-44.0007, -12.2983) knots 0 0 0 0 0.019923 0.019923 0.039846 0.039846 0.059769 0.059769 0.079691 0.079691 0.099614 0.099614 0.117812 0.117812 0.117812 0.117812
  line L76 (-25.9981, -13.5921) -> (-33.2388, -16.9993)
  spline S254 degree 5 poles (-42.826, -15.9134) (-42.8273, -15.9146) (-42.8403, -15.9271) (-42.8649, -15.9508) (-42.9012, -15.9859) (-42.9491, -16.0325) (-43.0071, -16.0895) (-43.065, -16.1468) (-43.1226, -16.2044) (-43.1801, -16.2623) (-43.2374, -16.3206) (-43.2945, -16.3791) (-43.3514, -16.4379) (-43.4081, -16.497) (-43.4646, -16.5564) (-43.521, -16.6161) (-43.5772, -16.6761) (-43.6332, -16.7364) (-43.689, -16.7969) (-43.7446, -16.8578) (-43.8, -16.9189) (-43.8553, -16.9803) (-43.8993, -17.0296) (-43.9323, -17.0668) (-43.9542, -17.0916) (-43.9652, -17.104) knots 0.712736 0.712736 0.712736 0.712736 0.712736 0.712736 0.714286 0.728571 0.742857 0.757143 0.771429 0.785714 0.8 0.814286 0.828571 0.842857 0.857143 0.871429 0.885714 0.9 0.914286 0.928571 0.942857 0.957143 0.971429 0.985714 1 1 1 1 1 1
  arc A161 (-37.1877, -1.1626) -> (-37.0691, -3.2831) centre (0.7975, -0.1016) ccw
  arc A162 (-43.9652, -17.104) -> (-43.7577, -17.628) centre (0, 0) ccw
  spline S255 degree 5 poles (-40.4939, -21.1555) (-40.495, -21.1568) (-40.5063, -21.1708) (-40.5278, -21.1974) (-40.5594, -21.2368) (-40.601, -21.289) (-40.6514, -21.3528) (-40.7016, -21.4169) (-40.7516, -21.4813) (-40.8014, -21.546) (-40.8509, -21.6109) (-40.9002, -21.6762) (-40.9493, -21.7417) (-40.9982, -21.8074) (-41.0468, -21.8734) (-41.0953, -21.9397) (-41.1435, -22.0063) (-41.1915, -22.0731) (-41.2392, -22.1402) (-41.2868, -22.2075) (-41.3341, -22.2751) (-41.3812, -22.3429) (-41.4188, -22.3974) (-41.4468, -22.4383) (-41.4655, -22.4657) (-41.4748, -22.4794) knots 0.712736 0.712736 0.712736 0.712736 0.712736 0.712736 0.714286 0.728571 0.742857 0.757143 0.771429 0.785714 0.8 0.814286 0.828571 0.842857 0.857143 0.871429 0.885714 0.9 0.914286 0.928571 0.942857 0.957143 0.971429 0.985714 1 1 1 1 1 1
  line L77 (-24.096, -16.8441) -> (-30.8526, -21.1319)
  spline S256 degree 5 poles (-41.7423, -18.5711) (-41.7435, -18.5724) (-41.7557, -18.5856) (-41.7788, -18.6109) (-41.8128, -18.6481) (-41.8576, -18.6976) (-41.912, -18.7582) (-41.9661, -18.819) (-42.02, -18.8801) (-42.0738, -18.9415) (-42.1273, -19.0032) (-42.1806, -19.0652) (-42.2337, -19.1275) (-42.2866, -19.1901) (-42.3393, -19.2529) (-42.3918, -19.3161) (-42.4441, -19.3794) (-42.4962, -19.4431) (-42.5481, -19.5071) (-42.5997, -19.5713) (-42.6512, -19.6357) (-42.7025, -19.7005) (-42.7434, -19.7525) (-42.7739, -19.7916) (-42.7943, -19.8177) (-42.8044, -19.8308) knots 0.712736 0.712736 0.712736 0.712736 0.712736 0.712736 0.714286 0.728571 0.742857 0.757143 0.771429 0.785714 0.8 0.814286 0.828571 0.842857 0.857143 0.871429 0.885714 0.9 0.914286 0.928571 0.942857 0.957143 0.971429 0.985714 1 1 1 1 1 1
  spline S257 degree 5 poles (-47.1742, -0.2818) (-47.1594, -0.2893) (-47.1299, -0.3043) (-47.0856, -0.3267) (-47.0264, -0.3563) (-46.9525, -0.3931) (-46.8784, -0.4295) (-46.8043, -0.4656) (-46.7302, -0.5013) (-46.6559, -0.5368) (-46.5816, -0.5719) (-46.5072, -0.6066) (-46.4328, -0.641) (-46.3583, -0.6751) (-46.2837, -0.7089) (-46.2091, -0.7423) (-46.1344, -0.7753) (-46.0596, -0.808) (-45.9848, -0.8404) (-45.9099, -0.8723) (-45.835, -0.904) (-45.7734, -0.9297) (-45.7267, -0.9489) (-45.695, -0.9619) (-45.6784, -0.9687) (-45.6768, -0.9694) knots -1 -1 -1 -1 -1 -1 -0.985714 -0.971429 -0.957143 -0.942857 -0.928571 -0.914286 -0.9 -0.885714 -0.871429 -0.857143 -0.842857 -0.828571 -0.814286 -0.8 -0.785714 -0.771429 -0.757143 -0.742857 -0.728571 -0.714286 -0.712736 -0.712736 -0.712736 -0.712736 -0.712736 -0.712736
  line L78 (-29.0826, -2.7806) -> (-37.0691, -3.2831)
  arc A163 (-46.3914, -8.5628) -> (-46.2858, -9.1163) centre (0, 0) ccw
  spline S258 degree 3 poles (-41.7423, -18.5711) (-41.6974, -18.5222) (-41.6624, -18.465) (-41.6164, -18.3404) (-41.6058, -18.2742) (-41.6106, -18.1414) (-41.6259, -18.0762) (-41.6807, -17.9552) (-41.7196, -17.9006) (-41.8162, -17.8095) (-41.873, -17.7738) (-41.9916, -17.7282) (-42.0517, -17.7167) (-42.1123, -17.7161) knots 0 0 0 0 0.019923 0.019923 0.039846 0.039846 0.059769 0.059769 0.079691 0.079691 0.099614 0.099614 0.117812 0.117812 0.117812 0.117812
  arc A164 (-42.8044, -19.8308) -> (-42.5645, -20.3407) centre (0, 0) ccw
  arc A165 (-36.7552, -5.9151) -> (-36.3717, -8.0039) centre (0.7975, -0.1016) ccw
  arc A166 (-26.7765, -11.9199) -> (-25.9981, -13.5921) centre (0.7975, -0.1016) ccw
  arc A167 (-34.1296, -15.0714) -> (-33.2388, -16.9993) centre (0.7975, -0.1016) ccw
  line L79 (-22.9712, -18.406) -> (-29.3095, -23.2871)
  spline S259 degree 5 poles (-45.4381, -4.7631) (-45.4396, -4.7639) (-45.4553, -4.7728) (-45.4851, -4.7896) (-45.5289, -4.8146) (-45.5869, -4.8478) (-45.6572, -4.8886) (-45.7275, -4.9297) (-45.7977, -4.9712) (-45.8678, -5.013) (-45.9377, -5.0551) (-46.0076, -5.0976) (-46.0774, -5.1404) (-46.147, -5.1836) (-46.2165, -5.2271) (-46.286, -5.2709) (-46.3553, -5.315) (-46.4245, -5.3595) (-46.4936, -5.4042) (-46.5626, -5.4493) (-46.6315, -5.4947) (-46.7003, -5.5405) (-46.7552, -5.5773) (-46.7964, -5.6051) (-46.8238, -5.6236) (-46.8375, -5.6329) knots 0.712736 0.712736 0.712736 0.712736 0.712736 0.712736 0.714286 0.728571 0.742857 0.757143 0.771429 0.785714 0.8 0.814286 0.828571 0.842857 0.857143 0.871429 0.885714 0.9 0.914286 0.928571 0.942857 0.957143 0.971429 0.985714 1 1 1 1 1 1
  spline S260 degree 3 poles (-45.4381, -4.7631) (-45.3802, -4.7304) (-45.3293, -4.6868) (-45.2471, -4.5825) (-45.2165, -4.5229) (-45.18, -4.3952) (-45.1744, -4.3283) (-45.1891, -4.1963) (-45.2093, -4.1324) (-45.273, -4.0159) (-45.316, -3.9644) (-45.4147, -3.8844) (-45.4683, -3.8549) (-45.5258, -3.8356) knots 0 0 0 0 0.019923 0.019923 0.039846 0.039846 0.059769 0.059769 0.079691 0.079691 0.099614 0.099614 0.117812 0.117812 0.117812 0.117812
  arc A168 (-41.4748, -22.4794) -> (-41.2033, -22.9733) centre (0, 0) ccw
  spline S261 degree 5 poles (-44.7782, -14.8456) (-44.7619, -14.8482) (-44.7291, -14.8533) (-44.6801, -14.8609) (-44.6147, -14.8709) (-44.533, -14.8829) (-44.4513, -14.8947) (-44.3697, -14.9061) (-44.2881, -14.9172) (-44.2065, -14.928) (-44.125, -14.9384) (-44.0436, -14.9485) (-43.9621, -14.9582) (-43.8807, -14.9676) (-43.7994, -14.9766) (-43.7181, -14.9853) (-43.6368, -14.9937) (-43.5556, -15.0017) (-43.4745, -15.0093) (-43.3934, -15.0166) (-43.3123, -15.0235) (-43.2458, -15.0289) (-43.1954, -15.0328) (-43.1613, -15.0354) (-43.1434, -15.0367) (-43.1416, -15.0368) knots -1 -1 -1 -1 -1 -1 -0.985714 -0.971429 -0.957143 -0.942857 -0.928571 -0.914286 -0.9 -0.885714 -0.871429 -0.857143 -0.842857 -0.828571 -0.814286 -0.8 -0.785714 -0.771429 -0.757143 -0.742857 -0.728571 -0.714286 -0.712736 -0.712736 -0.712736 -0.712736 -0.712736 -0.712736
  spline S262 degree 5 poles (-43.7407, -13.1929) (-43.7421, -13.1941) (-43.7558, -13.2057) (-43.7819, -13.2278) (-43.8203, -13.2606) (-43.871, -13.3041) (-43.9325, -13.3573) (-43.9938, -13.4109) (-44.055, -13.4647) (-44.116, -13.5189) (-44.1768, -13.5735) (-44.2375, -13.6283) (-44.298, -13.6834) (-44.3583, -13.7389) (-44.4185, -13.7946) (-44.4785, -13.8506) (-44.5383, -13.907) (-44.5979, -13.9636) (-44.6574, -14.0206) (-44.7168, -14.0778) (-44.7759, -14.1353) (-44.8349, -14.1931) (-44.882, -14.2396) (-44.9172, -14.2745) (-44.9406, -14.2979) (-44.9524, -14.3096) knots 0.712736 0.712736 0.712736 0.712736 0.712736 0.712736 0.714286 0.728571 0.742857 0.757143 0.771429 0.785714 0.8 0.814286 0.828571 0.842857 0.857143 0.871429 0.885714 0.9 0.914286 0.928571 0.942857 0.957143 0.971429 0.985714 1 1 1 1 1 1
  spline S263 degree 5 poles (-47.0634, -3.2433) (-47.0482, -3.2499) (-47.0178, -3.263) (-46.9721, -3.2825) (-46.9113, -3.3084) (-46.8351, -3.3405) (-46.759, -3.3722) (-46.6827, -3.4035) (-46.6065, -3.4346) (-46.5301, -3.4653) (-46.4538, -3.4956) (-46.3774, -3.5256) (-46.3009, -3.5553) (-46.2244, -3.5847) (-46.1479, -3.6137) (-46.0713, -3.6423) (-45.9947, -3.6706) (-45.918, -3.6985) (-45.8413, -3.7261) (-45.7646, -3.7533) (-45.6878, -3.7802) (-45.6247, -3.802) (-45.5769, -3.8183) (-45.5445, -3.8292) (-45.5274, -3.835) (-45.5258, -3.8356) knots -1 -1 -1 -1 -1 -1 -0.985714 -0.971429 -0.957143 -0.942857 -0.928571 -0.914286 -0.9 -0.885714 -0.871429 -0.857143 -0.842857 -0.828571 -0.814286 -0.8 -0.785714 -0.771429 -0.757143 -0.742857 -0.728571 -0.714286 -0.712736 -0.712736 -0.712736 -0.712736 -0.712736 -0.712736
  spline S264 degree 3 poles (-45.6475, -1.9006) (-45.5877, -1.8717) (-45.5342, -1.8313) (-45.4455, -1.7324) (-45.4113, -1.6748) (-45.3668, -1.5496) (-45.3571, -1.4833) (-45.3634, -1.3506) (-45.3796, -1.2855) (-45.4359, -1.1652) (-45.4755, -1.1112) (-45.569, -1.0251) (-45.6206, -0.9923) (-45.6768, -0.9694) knots 0 0 0 0 0.019923 0.019923 0.039846 0.039846 0.059769 0.059769 0.079691 0.079691 0.099614 0.099614 0.117812 0.117812 0.117812 0.117812
  arc A169 (-46.8375, -5.6329) -> (-46.7669, -6.192) centre (0, 0) ccw
  arc A170 (-29.1908, -0.9393) -> (-29.0826, -2.7806) centre (0.7975, -0.1016) ccw
  line L80 (-28.0403, -8.3707) -> (-35.7304, -10.5758)
  spline S265 degree 3 poles (-45.0493, -7.6067) (-44.9937, -7.5705) (-44.9456, -7.5238) (-44.87, -7.4146) (-44.8433, -7.3531) (-44.8149, -7.2234) (-44.8135, -7.1563) (-44.8365, -7.0255) (-44.8606, -6.963) (-44.9315, -6.8507) (-44.9776, -6.802) (-45.0812, -6.7283) (-45.1365, -6.7023) (-45.1951, -6.6866) knots 0 0 0 0 0.019923 0.019923 0.039846 0.039846 0.059769 0.059769 0.079691 0.079691 0.099614 0.099614 0.117812 0.117812 0.117812 0.117812
  spline S266 degree 3 poles (-39.0856, -23.6563) (-39.0471, -23.6022) (-39.0196, -23.541) (-38.9896, -23.4117) (-38.9874, -23.3447) (-39.0087, -23.2136) (-39.0321, -23.1507) (-39.1016, -23.0376) (-39.1471, -22.9883) (-39.2544, -22.91) (-39.3152, -22.8817) (-39.4386, -22.8514) (-39.4996, -22.8475) (-39.5598, -22.8544) knots 0 0 0 0 0.019923 0.019923 0.039846 0.039846 0.059769 0.059769 0.079691 0.079691 0.099614 0.099614 0.117812 0.117812 0.117812 0.117812
  line L81 (-27.4777, -10.1273) -> (-35.0882, -12.6001)
  line L82 (-28.8493, -4.6912) -> (-36.7552, -5.9151)
  spline S267 degree 5 poles (-46.7669, -6.192) (-46.7513, -6.1976) (-46.7201, -6.2088) (-46.6733, -6.2255) (-46.611, -6.2475) (-46.533, -6.2747) (-46.455, -6.3015) (-46.3769, -6.328) (-46.2988, -6.3542) (-46.2207, -6.3801) (-46.1426, -6.4056) (-46.0645, -6.4307) (-45.9863, -6.4556) (-45.9081, -6.48) (-45.8299, -6.5042) (-45.7517, -6.5279) (-45.6734, -6.5514) (-45.5952, -6.5744) (-45.5169, -6.5972) (-45.4386, -6.6195) (-45.3603, -6.6415) (-45.2959, -6.6593) (-45.2472, -6.6725) (-45.2142, -6.6815) (-45.1968, -6.6861) (-45.1951, -6.6866) knots -1 -1 -1 -1 -1 -1 -0.985714 -0.971429 -0.957143 -0.942857 -0.928571 -0.914286 -0.9 -0.885714 -0.871429 -0.857143 -0.842857 -0.828571 -0.814286 -0.8 -0.785714 -0.771429 -0.757143 -0.742857 -0.728571 -0.714286 -0.712736 -0.712736 -0.712736 -0.712736 -0.712736 -0.712736